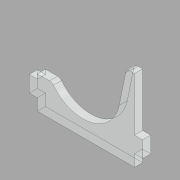
# Autodesk Inventor part: 104.003.01_Endanschlag_Flasche
Saved by Autodesk Inventor 2021 (Build 250183000, 183)
## iProperties
Created: 2021-02-19
Part Number: 104.003.01_Endanschlag_Flasche
Material: Generic
Document SubType Name: Modeling
Designer: work_CAD_TwinCAT
Density: 1 g/cm^3
Appearance: Default
Author: work_CAD_TwinCAT
Autodesk Inventor part; units mm, degrees
ref_plane "YZ Plane" through (0, 0, 0) normal (1, 0, 0) x (0, 1, 0)
ref_plane "XZ Plane" through (0, 0, 0) normal (0, 1, 0) x (-1, 0, 0)
ref_plane "XY Plane" through (0, 0, 0) normal (0, 0, 1) x (1, 0, 0)
sketch "Sketch1" plane through (0, 0, 0) normal (0, 0, 1) x (1, 0, 0)
  arc A0 (-18.9737, -13) -> (22.5323, -4.6147) centre (0, 0) ccw
  circle A1 centre (0, 0) radius 23 construction
  line L0 (-28, 0) -> (-28, -39.6186) construction
  line L1 (-18.9737, -13) -> (-28, -13)
  line L2 (-28, -13) -> (-28, -15.8)
  line L3 (-28, -15.8) -> (-33, -15.8)
  line L4 (-33, -15.8) -> (-33, -25.8)
  line L5 (37, -25.8) -> (37, -15.8)
  line L6 (37, -15.8) -> (32, -15.8)
  line L7 (32, -15.8) -> (32, 17.2)
  line L8 (-33, -25.8) -> (-28, -25.8)
  line L9 (-28, -33) -> (-28, -25.8)
  line L10 (-28, -33) -> (32, -33)
  line L11 (32, -33) -> (32, -25.8)
  line L12 (32, -25.8) -> (37, -25.8)
  line L13 (0, 0) -> (-28, 0) construction
  line L14 (22.5323, -4.6147) -> (27, 17.2)
  line L15 (27, 17.2) -> (32, 17.2)
  dimension "d0" = 46
  dimension "d1" = 15.8
  dimension "d2" = 13
  dimension "d3" = 5
  dimension "d4" = 5
  dimension "d5" = 10
  dimension "d6" = 60
  dimension "d7" = 33
  dimension "d10" = 33
  dimension "d13" = 28
  dimension "d14" = 5
  constraints: 32 end point, 6 perpendicular, 6 point on line, 4 horizontal, 3 vertical, 2 coincident, 2 collinear, 2 point on circle, 1 centre point, 1 tangent, 4 other
  measures "d1" distance from line of L3 L0.start
  measures "d2" distance from line of L0.start L1
  measures "d3" distance of L2.end L3.end
  measures "d4" distance of L5.end L6.end
  measures "d5" distance of L3.end L4.end
  measures "d6" distance between parallel lines of L7 L0
  measures "d7" distance of L6.end L7.end
  measures "d10" distance from line of L13.start L10
  measures "d13" distance from line of L13.start L0
  measures "d14" distance of L14.end L7.end
extrude "Extrusion1" add sketch "Sketch1" along normal blind 5
fillet "Fillet1" radius 3 2 edges at (-18.9737, -13, 2.5) (27, 17.2, 2.5)
equation "\"d4\" = d3"
body "Solid1"
